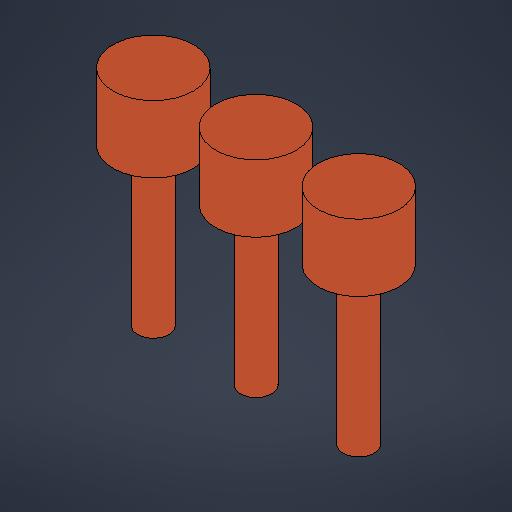
# Autodesk Inventor part: Pogo_Pin1
Saved by Autodesk Inventor 2026 (Build 300175000, 175)
## iProperties
Created: 2025-04-17
Part Number: Pogo_Pin1
Material: Copper
Document SubType Name: Modeling
Designer: ct_vi
Density: 8.94 g/cm^3
Appearance: Copper - Satin
Author: ct_vi
Autodesk Inventor part; units mm, degrees
ref_plane "YZ Plane" through (0, 0, 0) normal (1, 0, 0) x (0, 1, 0)
ref_plane "XZ Plane" through (0, 0, 0) normal (0, 1, 0) x (-1, 0, 0)
ref_plane "XY Plane" through (0, 0, 0) normal (0, 0, 1) x (1, 0, 0)
sketch "Sketch1" plane through (0, 0, 0) normal (0, 1, 0) x (-1, 0, 0)
  line L0 (-5.4, 3.15) -> (5.4, 3.15)
  line L1 (8.55, 0) -> (8.55, 0)
  line L2 (5.4, -3.15) -> (-5.4, -3.15)
  line L3 (-8.55, 0) -> (-8.55, 0)
  line L4 (-8.55, 3.15) -> (8.55, -3.15) construction
  line L5 (8.55, 3.15) -> (-8.55, -3.15) construction
  arc A0 (8.55, 0) -> (5.4, 3.15) centre (5.4, 0) ccw
  arc A1 (5.4, -3.15) -> (8.55, 0) centre (5.4, 0) ccw
  arc A2 (-5.4, 3.15) -> (-8.55, 0) centre (-5.4, 0) ccw
  arc A3 (-8.55, 0) -> (-5.4, -3.15) centre (-5.4, 0) ccw
  line L6 (5.4, 2.3494) -> (-5.4, 2.3494)
  line L7 (-7.75, -0.0006) -> (-7.75, 0.0006)
  line L8 (-5.4, -2.3494) -> (5.4, -2.3494)
  line L9 (7.75, 0.0006) -> (7.75, -0.0006)
  line L10 (7.75, 2.3494) -> (-7.75, -2.3494) construction
  line L11 (-7.75, 2.3494) -> (7.75, -2.3494) construction
  arc A4 (-5.4, 2.3494) -> (-7.75, -0.0006) centre (-5.4, -0.0006) ccw
  arc A5 (-7.75, 0.0006) -> (-5.4, -2.3494) centre (-5.4, 0.0006) ccw
  arc A6 (7.75, -0.0006) -> (5.4, 2.3494) centre (5.4, -0.0006) ccw
  arc A7 (5.4, -2.3494) -> (7.75, 0.0006) centre (5.4, 0.0006) ccw
  circle A8 centre (5.4, 0.0006) radius 1.5
  circle A9 centre (-5.4, 0.0006) radius 1.5
  circle A10 centre (2.3, 0) radius 0.9
  circle A11 centre (0, 0) radius 0.9
  circle A12 centre (-2.3, 0) radius 0.9
  circle A13 centre (2.3, 0) radius 0.35
  circle A14 centre (0, 0) radius 0.35
  circle A15 centre (-2.3, 0) radius 0.35
  point P0 (0, 0)
  dimension "d0" = 17.1
  dimension "d1" = 6.3
  dimension "d2" = 3.15
  dimension "d3" = 0.801
  dimension "d4" = 0.8
  dimension "d5" = 2.35
  dimension "d6" = 3
  dimension "d7" = 3
  dimension "d8" = 1.8
  dimension "d9" = 1.8
  dimension "d10" = 1.8
  dimension "d11" = 4.6
  dimension "d12" = 0.7
  dimension "d13" = 0.7
  dimension "d14" = 0.7
  constraints: 24 end point, 16 centre point, 16 point on circle, 16 point on line, 16 tangent, 6 coincident, 6 equal radius, 4 midpoint, 4 parallel, 2 horizontal, 2 perpendicular
  measures "d0" distance of L4.end L5.end
  measures "d1" distance of L5.start L4.end
  measures "d2" radius of A0
  measures "d4" distance from line of L3.end L7
  measures "d5" radius of A4
  measures "d6" diameter of A8
  measures "d7" diameter of A9
  measures "d8" diameter of A10
  measures "d9" diameter of A11
  measures "d10" diameter of A12
  measures "d11" distance of A12.centre A10.centre
  measures "d12" diameter of A13
  measures "d13" diameter of A14
  measures "d14" diameter of A15
extrude "Extrusion1" add sketch "Sketch1" along normal blind 2 and the other way blind 1.5 contours A13 | A14 | A15
sketch "Sketch2" plane through (-2.3, 2, 0) normal (0, 1, 0) x (1, 0, 0)
  circle A0 centre (0, 0) radius 0.9
  circle A1 centre (2.3, 0) radius 0.9
  line L0 (2.3, 0) -> (4.6, 0)
  circle A2 centre (4.6, 0) radius 0.9
  dimension "d21" = 1.8
  dimension "d22" = 1.8
  dimension "d23" = 2.3
  dimension "d24" = 1.8
  dimension "d25" = 2.3
  constraints: 3 centre point, 2 coincident, 2 end point, 1 horizontal
  measures "d21" diameter of A0
  measures "d22" diameter of A1
  measures "d23" distance of L0.start L0.end
  measures "d24" diameter of A2
  measures "d25" distance of point (2.3, 0) A0.centre
extrude "Extrusion2" add sketch "Sketch2" along normal blind 1.5
body "Solid1"
